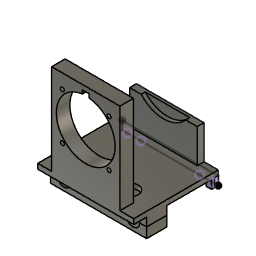
Motor support v21 (Autodesk Fusion 360 design; units mm, degrees)
Autodesk Fusion 360 part; units mm, degrees
sketch "Support base" plane through (0, 0, 0) normal (0, 1, 0) x (1, 0, 0)
  line L0 (0, 0) -> (0, -20)
  line L1 (142, 0) -> (142, -20)
  line L2 (0, -20) -> (142, -20)
  line L3 (0, 0) -> (142, 0)
  dimension "d18" = 20
  dimension "d32" = 142
  constraint coincident L0.start L3.start
  constraint equal L0 L1
  constraint perpendicular L1 L2
  constraint perpendicular L1 L3
  constraint equal L2 L3
  constraint horizontal L2
  measures "d18" distance of L0.start L0.end
  measures "d32" distance of L0.end L1.end
extrude "Extrude1" add sketch "Support base" along normal blind 125 makes body 1
sketch "Support screw 1" plane through (0, 0, 20) normal (0, 0, 1) x (-1, 0, 0)
  line L0 (0, 0) -> (-142, 0)
  line L1 (-142, 0) -> (-142, -125)
  line L2 (-142, -125) -> (0, -125)
  line L3 (0, -125) -> (0, 0)
  line L4 (0, 0) -> (-40, 0)
  line L5 (-40, 0) -> (-40, -34)
  circle A0 centre (-40, -34) radius 12.5
  line L6 (-142, 0) -> (-102, 0)
  line L7 (-102, 0) -> (-102, -34)
  circle A1 centre (-102, -34) radius 12.5
  dimension "d36" = 34
  dimension "d37" = 25
  dimension "d72" = 40
  constraint coincident L0.start L3.end
  constraint perpendicular L3 L4
  constraint perpendicular L4 L5
  constraint coincident L5.end A0.centre
  constraint coincident L0.end L1.start
  constraint perpendicular L1 L6
  constraint perpendicular L0 L7
  constraint coincident L7.end A1.centre
  constraint equal L4 L6
  constraint equal L5 L7
  constraint equal A0 A1
  measures "d36" distance of L4.end L5.end
  measures "d37" diameter of A0
  measures "d72" distance of L0.start L4.end
extrude "Extrude2" cut sketch "Support screw 1" against normal blind 7 contours A0 | A1 bodies 1
sketch "Support screw 2" plane through (0, 0, 13) normal (0, 0, 1) x (-1, 0, 0)
  circle A0 centre (-40, -34) radius 12.5
  line L0 (0, 0) -> (-40, 0)
  line L1 (-40, 0) -> (-40, -34)
  circle A1 centre (-40, -34) radius 4
  circle A2 centre (-102, -34) radius 4
  line L2 (-142, 0) -> (-102, 0)
  line L3 (-102, 0) -> (-102, -34)
  point P0 (-142, 0)
  dimension "d43" = 40
  dimension "d44" = 34
  dimension "d45" = 8
  constraint coincident L0.start origin
  constraint horizontal L0
  constraint perpendicular L0 L1
  constraint coincident A0.centre L1.end
  constraint horizontal L2
  constraint perpendicular L2 L3
  constraint coincident A2.centre L3.end
  constraint equal L0 L2
  constraint equal L1 L3
  constraint coincident P0 L2.start
  constraint equal A1 A2
  measures "d43" distance of L0.start L0.end
  measures "d44" distance of L0.end A0.centre
  measures "d45" diameter of A1
extrude "Extrude3" cut sketch "Support screw 2" against normal blind 20 contours A1 | A2 bodies 1
sketch "Support front" plane through (0, 0, 0) normal (0, -1, 0) x (1, 0, 0)
  line L0 (0, 20) -> (0, 0)
  line L1 (20.5, 154) -> (121.5, 154)
  line L2 (121.5, 154) -> (121.5, 20)
  line L3 (121.5, 20) -> (20.5, 20)
  line L4 (20.5, 20) -> (20.5, 154)
  line L5 (0, 20) -> (142, 20)
  line L6 (20.5, 20) -> (0, 20)
  line L7 (121.5, 20) -> (142, 20)
  line L8 (30, 139.5) -> (112, 139.5) construction
  line L9 (112, 139.5) -> (112, 57.5) construction
  line L10 (112, 57.5) -> (30, 57.5) construction
  line L11 (30, 57.5) -> (30, 139.5) construction
  line L12 (71, 139.5) -> (71, 57.5) construction
  line L13 (30, 98.5) -> (112, 98.5) construction
  line L14 (27.5, 142) -> (114.5, 142) construction
  line L15 (114.5, 142) -> (114.5, 55) construction
  line L16 (114.5, 55) -> (27.5, 55) construction
  line L17 (27.5, 55) -> (27.5, 142) construction
  line L18 (71, 142) -> (71, 55) construction
  line L19 (114.5, 98.5) -> (27.5, 98.5) construction
  line L20 (27.5, 142) -> (20.5, 142) construction
  line L21 (27.5, 142) -> (27.5, 154) construction
  line L22 (114.5, 142) -> (121.5, 142) construction
  line L23 (71, 142) -> (71, 147) construction
  line L24 (71, 147) -> (71, 154) construction
  line L25 (66, 147) -> (76, 147)
  line L26 (76, 147) -> (76, 141.7117)
  line L27 (66, 147) -> (66, 141.7117)
  arc A0 (66, 141.7117) -> (76, 141.7117) centre (71, 98.5) ccw
  line L28 (0, 0) -> (142, 0)
  circle A1 centre (36.5, 133) radius 3
  circle A2 centre (105.5, 133) radius 3
  circle A3 centre (36.5, 64) radius 3
  circle A4 centre (105.5, 64) radius 3
  line L29 (36.5, 133) -> (36.5, 139.5) construction
  line L30 (36.5, 64) -> (36.5, 57.5) construction
  line L31 (105.5, 64) -> (105.5, 57.5) construction
  line L32 (105.5, 133) -> (105.5, 139.5) construction
  line L33 (36.5, 133) -> (30, 133) construction
  line L34 (36.5, 64) -> (30, 64) construction
  line L35 (105.5, 64) -> (112, 64) construction
  line L36 (105.5, 133) -> (112, 133) construction
  point P0 (142, 20)
  dimension "d75" = 87
  dimension "d124" = 87
  dimension "d125" = 7
  dimension "d126" = 35
  dimension "d127" = 82
  dimension "d132" = 5
  dimension "d134" = 10
  dimension "d151" = 6
  dimension "d155" = 101
  dimension "d200" = 6.5
  dimension "d201" = 6.5
  constraint horizontal L1
  constraint vertical L2
  constraint horizontal L3
  constraint vertical L4
  constraint collinear L3 L5
  constraint coincident L0.start L5.start
  constraint coincident P0 L5.end
  constraint equal L6 L7
  constraint horizontal L8
  constraint vertical L9
  constraint horizontal L10
  constraint vertical L11
  constraint midpoint L8 L12.start
  constraint midpoint L10 L12.end
  constraint midpoint L11 L13.start
  constraint midpoint L9 L13.end
  constraint midpoint A0.centre L13
  constraint equal L12 L13
  constraint horizontal L14
  constraint vertical L15
  constraint horizontal L16
  constraint vertical L17
  constraint midpoint L14 L18.start
  constraint midpoint L16 L18.end
  constraint midpoint L15 L19.start
  constraint midpoint L17 L19.end
  constraint equal L18 L19
  constraint midpoint A0.centre L19
  constraint coincident L4 L20.end
  constraint perpendicular L4 L20
  constraint coincident L1 L21.end
  constraint perpendicular L1 L21
  constraint coincident L2 L22.end
  constraint perpendicular L2 L22
  constraint equal L20 L22
  constraint perpendicular L14 L23
  constraint midpoint L1 L24.end
  constraint perpendicular L23 L25
  constraint midpoint L23.end L25
  constraint perpendicular L25 L26
  constraint perpendicular L14 L27
  constraint equal L20 L24
  constraint coincident A1.centre L29.start
  constraint coincident L8 L29.end
  constraint perpendicular L8 L29
  constraint equal A1 A2
  constraint equal A2 A4
  constraint equal A3 A4
  constraint coincident A3.centre L30.start
  constraint coincident L10 L30.end
  constraint perpendicular L10 L30
  constraint coincident A4.centre L31.start
  constraint coincident L10 L31.end
  constraint perpendicular L10 L31
  constraint coincident A2.centre L32.start
  constraint coincident L8 L32.end
  constraint perpendicular L8 L32
  constraint equal L31 L32
  constraint equal L30 L31
  constraint equal L29 L30
  constraint coincident L11 L33.end
  constraint perpendicular L11 L33
  constraint coincident L11 L34.end
  constraint perpendicular L11 L34
  constraint coincident L9 L35.end
  constraint perpendicular L9 L35
  constraint coincident L9 L36.end
  constraint perpendicular L9 L36
  constraint equal L33 L34
  constraint equal L34 L35
  constraint equal L35 L36
  measures "d75" diameter of A0
  measures "d124" distance of L14.start L16.end
  measures "d125" distance of L14.start L20.end
  measures "d126" distance of L3 L16
  measures "d127" distance of L8.start L10.end
  measures "d132" distance of L18.start L23.end
  measures "d134" distance of L25.start L25.end
  measures "d151" diameter of A1
  measures "d155" distance of L1.start L1.end
  measures "d200" distance of A1.centre L29.end
  measures "d201" distance of A1.centre L33.end
extrude "Extrude6" add sketch "Support front" along normal blind 0 and the other way blind 20 bodies 1
sketch "Support back" plane through (0, 125, 0) normal (0, 1, 0) x (-1, 0, 0)
  line L0 (0, 0) -> (0, 20)
  line L1 (0, 20) -> (-142, 20)
  line L2 (-142, 20) -> (-142, 0)
  line L3 (-121, 20) -> (-21, 20)
  line L4 (-21, 20) -> (-21, 70)
  line L5 (-121, 70) -> (-121, 20)
  line L6 (-121, 70) -> (-21, 70)
  line L7 (-142, 0) -> (0, 0)
  line L8 (-121, 20) -> (-142, 20) construction
  line L9 (-21, 20) -> (0, 20) construction
  dimension "d108" = 50
  dimension "d157" = 100
  constraint horizontal L3
  constraint vertical L4
  constraint vertical L5
  constraint coincident L1 L3.start
  constraint perpendicular L4 L6
  constraint coincident L1.end L2.start
  constraint coincident L0.end L1.start
  constraint perpendicular L0 L9
  constraint equal L8 L9
  measures "d108" distance of L3.start L5.start
  measures "d157" distance of L4 L5
extrude "Extrude7" add sketch "Support back" against normal blind 10 contours L1 L3 L4 L5 L6 bodies 1
sketch "Motor placement" plane through (0, 0, 0) normal (0, -1, 0) x (1, 0, 0)
  line L0 (121.5, 20) -> (121.5, 154)
  line L1 (121.5, 154) -> (20.5, 154)
  line L2 (20.5, 154) -> (20.5, 20)
  line L3 (0, 20) -> (0, 0)
  line L4 (142, 0) -> (142, 20)
  line L5 (142, 20) -> (121.5, 20)
  line L6 (20.5, 20) -> (0, 20)
  circle A0 centre (71, 98.5) radius 43.5
  line L7 (27.5, 142) -> (114.5, 142) construction
  line L8 (114.5, 142) -> (114.5, 55) construction
  line L9 (114.5, 55) -> (27.5, 55) construction
  line L10 (27.5, 55) -> (27.5, 142) construction
  line L11 (30, 139.5) -> (112, 139.5) construction
  line L12 (112, 139.5) -> (112, 57.5) construction
  line L13 (112, 57.5) -> (30, 57.5) construction
  line L14 (30, 57.5) -> (30, 139.5) construction
  line L15 (71, 142) -> (71, 55) construction
  line L16 (27.5, 98.5) -> (114.5, 98.5) construction
  line L17 (71, 139.5) -> (71, 57.5) construction
  line L18 (30, 98.5) -> (112, 98.5) construction
  line L19 (27.5, 142) -> (20.5, 142) construction
  line L20 (114.5, 142) -> (121.5, 142) construction
  arc A1 (66, 141.7117) -> (76, 141.7117) centre (71, 98.5) ccw
  line L21 (0, 0) -> (142, 0)
  circle A2 centre (105.5, 64) radius 3
  circle A3 centre (36.5, 64) radius 3
  circle A4 centre (36.5, 133) radius 3
  circle A5 centre (105.5, 133) radius 3
  dimension "d129" = 87
  dimension "d130" = 87
  dimension "d131" = 82
  dimension "d135" = 35
  constraint horizontal L7
  constraint vertical L8
  constraint horizontal L9
  constraint vertical L10
  constraint horizontal L11
  constraint vertical L12
  constraint horizontal L13
  constraint vertical L14
  constraint midpoint L7 L15.start
  constraint midpoint L9 L15.end
  constraint midpoint L10 L16.start
  constraint midpoint L8 L16.end
  constraint midpoint L11 L17.start
  constraint midpoint L13 L17.end
  constraint midpoint L14 L18.start
  constraint midpoint L12 L18.end
  constraint equal L15 L16
  constraint equal L17 L18
  constraint midpoint A0.centre L16
  constraint midpoint A0.centre L18
  constraint coincident L2 L19.end
  constraint perpendicular L2 L19
  constraint coincident L0 L20.end
  constraint perpendicular L0 L20
  constraint equal L19 L20
  measures "d129" diameter of A0
  measures "d130" distance of L7.start L9.end
  measures "d131" distance of L11.start L13.end
  measures "d135" distance of L6 L9
extrude "Extrude8" cut sketch "Motor placement" against normal blind 121 contours A0 A1 bodies 1
ref_plane "WorkPlane1" through (0, 19, 0) normal (0, 1, 0) x (0, 0, 1)
sketch "Bottom base" plane through (0, 19, 0) normal (0, 1, 0) x (1, 0, 0)
  line L0 (0, 0) -> (142, 0)
  line L1 (142, 0) -> (142, 15)
  line L2 (142, 15) -> (0, 15)
  line L3 (0, 15) -> (0, 0)
  dimension "d178" = 15
  dimension "d179" = 142
  constraint coincident L0.start L3.end
  constraint horizontal L0
  constraint perpendicular L0 L1
  constraint perpendicular L1 L2
  constraint perpendicular L0 L3
  measures "d178" distance of L0 L1.end
  measures "d179" distance of L0.start L0.end
extrude "Extrude9" add sketch "Bottom base" along normal blind 30 separate body makes body 2
sketch "Sketch17" plane through (0, 0, 0) normal (0, 0, 1) x (-1, 0, 0)
  line L0 (0, -19) -> (-142, -19)
  line L1 (-142, -19) -> (-142, -49)
  line L2 (-142, -49) -> (0, -49)
  line L3 (0, -49) -> (0, -19)
  line L4 (0, -19) -> (-40, -19) construction
  line L5 (-142, -19) -> (-102, -19) construction
  circle A0 centre (-40, -34) radius 4
  circle A1 centre (-102, -34) radius 4
  line L6 (-40, -19) -> (-40, -49) construction
  line L7 (-102, -19) -> (-102, -49) construction
  dimension "d184" = 40
  dimension "d186" = 8
  constraint coincident L0.start L3.end
  constraint coincident L0 L4.end
  constraint perpendicular L3 L4
  constraint coincident L0.end L1.start
  constraint coincident L0 L5.end
  constraint perpendicular L1 L5
  constraint equal L4 L5
  constraint equal A0 A1
  constraint coincident L2 L6.end
  constraint perpendicular L2 L6
  constraint coincident L2 L7.end
  constraint perpendicular L2 L7
  constraint midpoint A0.centre L6
  constraint midpoint A1.centre L7
  measures "d184" distance of L0.start L4.end
  measures "d186" diameter of A0
extrude "Extrude10" cut sketch "Sketch17" against normal blind 50 contours A0 | A1 bodies 2
sketch "Pipes front" plane through (0, 0, 0) normal (0, -1, 0) x (1, 0, 0)
  line L0 (66, 141.7117) -> (66, 147)
  line L1 (66, 147) -> (76, 147)
  line L2 (76, 147) -> (76, 141.7117)
  arc A0 (66, 141.7117) -> (76, 141.7117) centre (71, 98.5) ccw
  line L3 (20.5, 20) -> (0, 20)
  line L4 (0, 20) -> (0, 0)
  line L5 (142, 0) -> (142, 20)
  line L6 (142, 20) -> (121.5, 20)
  line L7 (121.5, 20) -> (121.5, 154)
  line L8 (121.5, 154) -> (20.5, 154)
  line L9 (20.5, 154) -> (20.5, 20)
  line L10 (0, 0) -> (10.5, 0) construction
  line L11 (30.5, 0) -> (111.5, 0) construction
  line L12 (131.5, 0) -> (142, 0) construction
  circle A1 centre (20.5, 0) radius 10
  circle A2 centre (121.5, 0) radius 10
  circle A3 centre (105.5, 64) radius 3
  circle A4 centre (36.5, 64) radius 3
  circle A5 centre (36.5, 133) radius 3
  circle A6 centre (105.5, 133) radius 3
  line L13 (10.5, 0) -> (30.5, 0) construction
  line L14 (111.5, 0) -> (131.5, 0) construction
  dimension "d163" = 81
  dimension "d189" = 20
  constraint coincident L4.end L10.start
  constraint coincident L5.start L12.end
  constraint perpendicular L5 L12
  constraint equal L10 L12
  constraint coincident L11.start A1
  constraint coincident L12.start A2
  constraint equal A1 A2
  constraint coincident L10.end A1
  constraint coincident L11.end A2
  constraint horizontal L10
  constraint horizontal L11
  constraint collinear L10 L11
  constraint midpoint A1.centre L13
  constraint midpoint A2.centre L14
  measures "d163" distance of L11.start L11.end
  measures "d189" diameter of A1
sketch "Pipes back" plane through (0, 125, 0) normal (0, 1, 0) x (-1, 0, 0)
  line L0 (0, 20) -> (-21, 20)
  line L1 (-142, 20) -> (-142, 0)
  line L2 (0, 0) -> (0, 20)
  line L3 (-142, 0) -> (-134.5, 0) construction
  line L4 (-114.5, 0) -> (-27.5, 0) construction
  line L5 (-7.5, 0) -> (0, 0) construction
  line L6 (-21, 20) -> (-21, 70)
  line L7 (-21, 70) -> (-121, 70)
  line L8 (-121, 70) -> (-121, 20)
  line L9 (-121, 20) -> (-142, 20)
  circle A0 centre (-124.5, 0) radius 10
  circle A1 centre (-17.5, 0) radius 10
  line L10 (-134.5, 0) -> (-114.5, 0) construction
  line L11 (-27.5, 0) -> (-7.5, 0) construction
  dimension "d164" = 87
  dimension "d190" = 20
  constraint coincident L1.end L3.start
  constraint perpendicular L1 L3
  constraint coincident L2.start L5.end
  constraint perpendicular L2 L5
  constraint equal L3 L5
  constraint coincident L4.start A0
  constraint coincident L5.start A1
  constraint equal A0 A1
  constraint coincident L3.end A0
  constraint coincident L4.end A1
  constraint horizontal L4
  constraint collinear L3 L4
  constraint collinear L1.end A0.centre A1.centre
  constraint midpoint A0.centre L10
  measures "d164" distance of L4.start L4.end
  measures "d190" diameter of A0
loft "Loft1" cut profiles "Pipes front", "Pipes back" section 1 contours A1 section 2 contours A1 bodies 1 2
loft "Loft2" cut profiles "Pipes front", "Pipes back" section 1 contours A2 section 2 contours A0 bodies 1 2
sketch "Sketch18" plane through (0, 125, 0) normal (0, 1, 0) x (-1, 0, 0)
  line L0 (-114.5, 0) -> (-27.5, 0)
  line L1 (-7.5, 0) -> (0, 0)
  line L2 (0, 0) -> (0, 20)
  line L3 (0, 20) -> (-21, 20)
  line L4 (-21, 20) -> (-21, 70)
  line L5 (-21, 70) -> (-121, 70)
  line L6 (-121, 70) -> (-121, 20)
  line L7 (-121, 20) -> (-142, 20)
  line L8 (-142, 20) -> (-142, 0)
  line L9 (-142, 0) -> (-134.5, 0)
  line L10 (-142, 0) -> (0, 0)
  line L11 (0, 0) -> (0, 12.5)
  line L12 (0, 12.5) -> (-142, 12.5)
  line L13 (-142, 12.5) -> (-142, 0)
  dimension "d202" = 12.5
  constraint horizontal L10
  constraint vertical L11
  constraint horizontal L12
  constraint vertical L13
  constraint coincident L2 L11.end
  constraint coincident L8.end L9.start
  measures "d202" distance of L10 L12
extrude "Extrude11" cut sketch "Sketch18" against normal blind 5 contours L0 L1 L2 L8 L9 L10 L11 L12 L13 bodies 1
extrude "Extrude12" cut sketch "Sketch18" against normal up to surface (66 mm away) from surface at -10 contours L0 L1 L2 L8 L9 L10 L11 L12 L13 bodies 1
extrude "Extrude13" cut sketch "Sketch18" against normal up to surface (19 mm away) from surface at -106 contours L0 L1 L2 L8 L9 L10 L11 L12 L13 bodies 1
fillet "Fillet1" [suppressed]
fillet "Fillet2" [suppressed]
equation "d18 = support_height"
equation "d32 = support_width"
equation "d33 = support_length"
equation "d36 = support_screw_ypos"
equation "d37 = support_screw_ring_radius"
equation "d41 = support_screw_ring_deepness"
equation "d43 = support_screw_xpos"
equation "d44 = support_screw_ypos"
equation "d45 = support_screw_radius"
equation "d72 = support_screw_xpos"
equation "d75 = motor_radius"
equation "d103 = support_front_thickness"
equation "d108 = support_back_height"
equation "d110 = support_back_thickness"
equation "d118 = -motor_length"
equation "d124 = motor_radius"
equation "d125 = motor_padding"
equation "d126 = motor_height_offset"
equation "d127 = motor_width"
equation "d129 = motor_radius"
equation "d130 = motor_radius"
equation "d131 = motor_width"
equation "d132 = motor_cable_height"
equation "d134 = motor_cable_width"
equation "d135 = motor_height_offset"
equation "support_screw_ring_radius = 2.5 cm"
equation "support_screw_xpos = 4 cm"
equation "support_screw_ypos = 3.4 cm"
equation "support_screw_radius = 0.8 cm"
equation "support_height = 2 cm"
equation "support_width = 14.2 cm"
equation "motor_radius = 8.7 cm"
equation "motor_width = 8.2 cm"
equation "motor_length = 12.1 cm"
equation "motor_plate_thickness = 0.5 cm"
equation "motor_height_offset = 3.5 cm"
equation "motor_padding = 0.7 cm"
equation "motor_screw_padding = 0.35 cm"
equation "motor_screw_diameter = 0.6 cm"
equation "d151 = motor_screw_diameter"
equation "motor_cable_height = 0.5 cm"
equation "motor_cable_width = 1 cm"
equation "support_back_height = motor_height_offset + 1.5 cm"
equation "support_back_width = 10 cm"
equation "d157 = support_back_width"
equation "pipe_diameter = 1.9 cm"
equation "pipe_front_separation = 8.2 cm" comment "Pipies are not parralels. Need to loft from one side to the other."
equation "pipe_back_separation = 8.8 cm" comment "Pipies are not parralels. Need to loft from one side to the other."
equation "d163 = pipe_front_separation - 2 * pipe_padding / 2"
equation "d164 = pipe_back_separation - 2 * pipe_padding / 2"
equation "pipe_padding = 0.1 cm"
equation "support_bottom_height = 1.5 cm"
equation "support_bottom_width = support_width"
equation "support_bottom_length = 3 cm"
equation "support_length = 12.5 cm"
equation "support_screw_ring_deepness = -0.7 cm"
equation "support_front_thickness = 2 cm"
equation "support_back_thickness = -1 cm"
equation "support_bottom_setback = support_screw_ypos - support_bottom_length / 2"
equation "d177 = support_bottom_setback"
equation "d178 = support_bottom_height"
equation "d179 = support_bottom_width"
equation "d182 = support_bottom_length"
equation "d184 = support_screw_xpos"
equation "d186 = support_screw_radius"
equation "d187 = -support_back_height"
equation "d189 = pipe_diameter + pipe_padding"
equation "d190 = pipe_diameter + pipe_padding"
equation "fillet_radius = 0.1 cm"
equation "d195 = fillet_radius"
equation "d197 = fillet_radius"
equation "d199 = fillet_radius"
equation "d200 = motor_screw_padding + motor_screw_diameter / 2"
equation "d201 = motor_screw_padding + motor_screw_diameter / 2"
equation "d202 = pipe_diameter / 2 + support_adjustment_height"
equation "support_adjustment_height = 0.3 cm"
